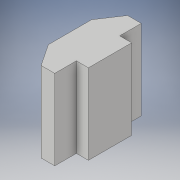
# Autodesk Inventor part: test_slot
Saved by Autodesk Inventor 2018 (Build 220112000, 112)
## iProperties
Created: 2020-03-14
Part Number: test_slot
Material: Generic
Document SubType Name: Modeling
Designer: natha
Density: 1 g/cm^3
Appearance: Default
Author: natha
Autodesk Inventor part; units mm, degrees
ref_plane "YZ Plane" through (0, 0, 0) normal (1, 0, 0) x (0, 1, 0)
ref_plane "XZ Plane" through (0, 0, 0) normal (0, 1, 0) x (-1, 0, 0)
ref_plane "XY Plane" through (0, 0, 0) normal (0, 0, 1) x (1, 0, 0)
sketch "Sketch1" plane through (0, 0, 0) normal (0, 1, 0) x (-1, 0, 0)
  line L0 (0, 0) -> (0, -5.4)
  line L1 (0, -5.4) -> (1.5, -5.4)
  line L2 (1.5, -5.4) -> (1.5, -8.1)
  line L3 (1.5, -8.1) -> (3.2, -8.1)
  line L4 (0, 0) -> (1.5, 0)
  line L5 (1.5, 0) -> (1.5, 2.7)
  line L6 (1.5, 2.7) -> (3.2, 2.7)
  line L7 (5, 0) -> (5, -5.4)
  line L8 (5, -5.4) -> (3.2, -8.1)
  line L9 (5, 0) -> (3.2, 2.7)
  dimension "d0" = 5.4
  dimension "d1" = 1.5
  dimension "d2" = 2.7
  dimension "d3" = 1.7
  dimension "d4" = 2.7
  dimension "d5" = 1.7
  dimension "d6" = 5
  constraints: 20 end point, 5 perpendicular, 2 vertical, 1 horizontal
  measures "d0" distance of L0.start L0.end
  measures "d1" distance of L0.end L1.end
  measures "d2" distance of L1.end L2.end
  measures "d3" distance of L2.end L3.end
  measures "d4" distance of L4.end L5.end
  measures "d5" distance of L5.end L6.end
  measures "d6" distance between parallel lines of L7 L0
extrude "Extrusion1" add sketch "Sketch1" along normal blind 10
body "Solid1"
